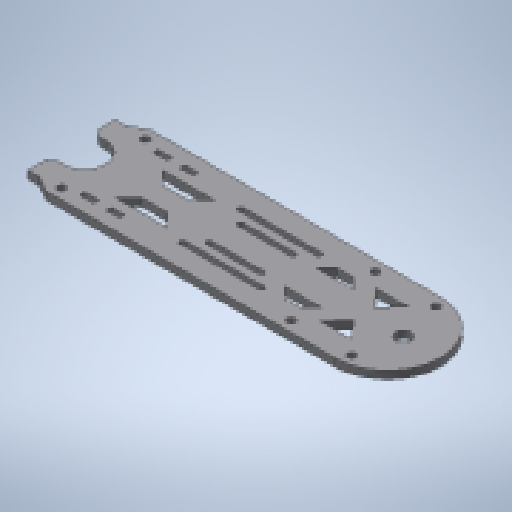
# Autodesk Inventor part: topplate.rev4
Saved by Autodesk Inventor 2025.2 (Build 292293000, 293)
## iProperties
Created: 2016-03-08
Part Number: topplate.rev4
Material: 一般
Document SubType Name: Modeling
Designer: 200288284
Density: 1 g/cm^3
Appearance: 默认值
Author: 200288284
Autodesk Inventor part; units mm, degrees
ref_plane "YZ Plane" through (0, 0, 0) normal (1, 0, 0) x (0, 1, 0)
ref_plane "XZ Plane" through (0, 0, 0) normal (0, 1, 0) x (-1, 0, 0)
ref_plane "XY Plane" through (0, 0, 0) normal (0, 0, 1) x (1, 0, 0)
sketch "Sketch1" plane through (0, 0, 0) normal (0, 1, 0) x (-1, 0, 0)
  line L0 (-71.934, -191.4381) -> (-71.9231, -191.4456)
  line L1 (19.6087, -153.4475) -> (19.6065, -153.4456)
  line L2 (-67.3897, -0.1562) -> (-37.3897, -0.1562)
  line L3 (-37.3897, 1.8438) -> (-67.3897, 1.8438)
  line L4 (-62.3897, -3.1562) -> (-42.3897, -3.1562)
  line L5 (-42.3897, -5.1562) -> (-62.3897, -5.1562)
  line L6 (-113.9275, -186.1817) -> (-113.9275, -186.2664)
  line L7 (-115.4443, -311.1974) -> (-115.4443, -311.1982)
  line L8 (-113.9275, -180.4456) -> (-113.9275, -180.5089)
  circle A0 centre (-110.3897, -10.1562) radius 3
  arc A1 (10.8743, -2.1562) -> (10.8743, -18.1562) centre (10.8743, -10.1562) ccw
  arc A2 (-42.3897, -5.1562) -> (-42.3897, -3.1562) centre (-42.3897, -4.1562) ccw
  arc A3 (-62.3897, -3.1562) -> (-62.3897, -5.1562) centre (-62.3897, -4.1562) ccw
  arc A4 (-67.3897, 1.8438) -> (-67.3897, -0.1562) centre (-67.3897, 0.8438) ccw
  arc A5 (-37.3897, -0.1562) -> (-37.3897, 1.8438) centre (-37.3897, 0.8438) ccw
  arc A6 (-104.3897, 9.8438) -> (-104.3897, -30.1562) centre (-104.3897, -10.1562) ccw
  line L9 (5.6103, 9.8438) -> (11.6725, 6.3438)
  line L10 (11.6725, 6.3438) -> (15.6725, 6.3438)
  line L11 (15.6725, 6.3438) -> (15.6725, -0.2278)
  line L12 (15.6725, -0.2278) -> (13.3743, -2.1562)
  line L13 (13.3743, -2.1562) -> (10.8743, -2.1562)
  line L14 (5.6103, 9.8438) -> (-104.3897, 9.8438)
  line L15 (-89.3897, 0.552) -> (-101.3897, 0.552)
  line L16 (-101.3897, 0.552) -> (-95.3897, -6.1562)
  line L17 (-95.3897, -6.1562) -> (-89.3897, 0.552)
  line L18 (-85.3897, -4.1562) -> (-81.3897, -0.1562)
  line L19 (-75.3897, -0.1562) -> (-71.3897, -4.1562)
  line L20 (-71.3897, -4.1562) -> (-85.3897, -4.1562)
  line L21 (-81.3897, -0.1562) -> (-75.3897, -0.1562)
  line L22 (-68.2196, -182.5089) -> (-68.232, -182.5206)
  line L23 (-104.3897, 9.8438) -> (-104.3897, -30.1562)
  line L24 (-104.3897, -10.1562) -> (10.8743, -10.1562)
  line L25 (-110.3897, -10.1562) -> (-104.3897, -10.1562)
  line L26 (10.8743, -2.1562) -> (10.8743, -18.1562)
  line L27 (5.6103, -30.1562) -> (11.6725, -26.6562)
  line L28 (11.6725, -26.6562) -> (15.6725, -26.6562)
  line L29 (15.6725, -26.6562) -> (15.6725, -20.0845)
  line L30 (15.6725, -20.0845) -> (13.3743, -18.1562)
  line L31 (13.3743, -18.1562) -> (10.8743, -18.1562)
  line L32 (5.6103, -30.1562) -> (-104.3897, -30.1562)
  line L33 (-2.3577, 2.8438) -> (-7.5577, 2.8438)
  line L34 (-7.5577, 2.8438) -> (-7.5577, 4.8438)
  line L35 (-2.3577, 4.8438) -> (-7.5577, 4.8438)
  line L36 (-2.3577, 2.8438) -> (-2.3577, 4.8438)
  line L37 (-12.3577, 2.8438) -> (-17.5577, 2.8438)
  line L38 (-17.5577, 2.8438) -> (-17.5577, 4.8438)
  line L39 (-12.3577, 4.8438) -> (-17.5577, 4.8438)
  line L40 (-12.3577, 2.8438) -> (-12.3577, 4.8438)
  line L41 (-46.7577, -10.1562) -> (-46.7577, 9.8438)
  line L42 (-2.3577, -23.1562) -> (-7.5577, -23.1562)
  line L43 (-7.5577, -23.1562) -> (-7.5577, -25.1562)
  line L44 (-2.3577, -25.1562) -> (-7.5577, -25.1562)
  line L45 (-2.3577, -23.1562) -> (-2.3577, -25.1562)
  line L46 (-12.3577, -23.1562) -> (-17.5577, -23.1562)
  line L47 (-17.5577, -23.1562) -> (-17.5577, -25.1562)
  line L48 (-12.3577, -25.1562) -> (-17.5577, -25.1562)
  line L49 (-12.3577, -23.1562) -> (-12.3577, -25.1562)
  circle A7 centre (3.6423, -25.1562) radius 1.55
  circle A8 centre (3.5423, 4.8438) radius 1.55
  circle A9 centre (-83.7577, 4.8438) radius 1.55
  circle A10 centre (-106.7577, 4.8438) radius 1.55
  circle A11 centre (-83.7577, -25.1562) radius 1.55
  circle A12 centre (-106.7577, -25.1562) radius 1.55
  line L50 (-62.3897, -17.1562) -> (-42.3897, -17.1562)
  line L51 (-42.3897, -15.1562) -> (-62.3897, -15.1562)
  line L52 (-67.3897, -20.1562) -> (-37.3897, -20.1562)
  line L53 (-37.3897, -22.1562) -> (-67.3897, -22.1562)
  arc A13 (-42.3897, -17.1562) -> (-42.3897, -15.1562) centre (-42.3897, -16.1562) ccw
  arc A14 (-62.3897, -15.1562) -> (-62.3897, -17.1562) centre (-62.3897, -16.1562) ccw
  arc A15 (-67.3897, -20.1562) -> (-67.3897, -22.1562) centre (-67.3897, -21.1562) ccw
  arc A16 (-37.3897, -22.1562) -> (-37.3897, -20.1562) centre (-37.3897, -21.1562) ccw
  line L54 (-89.3897, -20.8644) -> (-101.3897, -20.8644)
  line L55 (-101.3897, -20.8644) -> (-95.3897, -14.1562)
  line L56 (-95.3897, -14.1562) -> (-89.3897, -20.8644)
  line L57 (-85.3897, -16.1562) -> (-81.3897, -20.1562)
  line L58 (-75.3897, -20.1562) -> (-71.3897, -16.1562)
  line L59 (-71.3897, -16.1562) -> (-85.3897, -16.1562)
  line L60 (-81.3897, -20.1562) -> (-75.3897, -20.1562)
  line L61 (-29.7577, -1.1562) -> (-9.7577, -1.1562)
  line L62 (-9.7577, -1.1562) -> (-14.7577, -6.1562)
  line L63 (-14.7577, -6.1562) -> (-24.7577, -6.1562)
  line L64 (-24.7577, -6.1562) -> (-29.7577, -1.1562)
  line L65 (-29.7577, -19.1562) -> (-9.7577, -19.1562)
  line L66 (-9.7577, -19.1562) -> (-14.7577, -14.1562)
  line L67 (-14.7577, -14.1562) -> (-24.7577, -14.1562)
  line L68 (-24.7577, -14.1562) -> (-29.7577, -19.1562)
  dimension "d39" = 6
  dimension "d54" = 40
  dimension "d55" = 6
  dimension "d56" = 20
  dimension "d58" = 110
  dimension "d60" = 150
  dimension "d61" = 130
  dimension "d62" = 4
  dimension "d63" = 2.5
  dimension "d64" = 7
  dimension "d65" = 3
  dimension "d70" = 8
  dimension "d74" = 2
  dimension "d75" = 5.2
  dimension "d76" = 2
  dimension "d77" = 5.2
  dimension "d78" = 4.8
  dimension "d79" = 13
  dimension "d80" = 13
  dimension "d81" = 29.2
  dimension "d82" = 3.1
  dimension "d83" = 3.1
  dimension "d84" = 5.9
  dimension "d85" = 6
  dimension "d86" = 15
  dimension "d87" = 15
  dimension "d88" = 3.1
  dimension "d89" = 3.1
  dimension "d90" = 15
  dimension "d91" = 15
  dimension "d92" = 37
  dimension "d93" = 23
  dimension "d94" = 12
  dimension "d95" = 9
  dimension "d96" = 14
  dimension "d97" = 6
  dimension "d99" = 4
  dimension "d100" = 9
  dimension "d101" = 6
  dimension "d102" = 10
  dimension "d103" = 2
  dimension "d104" = 20
  dimension "d105" = 2
  dimension "d106" = 5
  dimension "d108" = 30
  dimension "d109" = 10
  dimension "d110" = 42
  dimension "d111" = 5
  dimension "d112" = 20
  dimension "d113" = 10
  dimension "d114" = 45
  dimension "d115" = 4
  dimension "d116" = 22
  constraints: 138 end point, 38 symmetric about line, 20 point on circle, 17 centre point, 8 horizontal, 8 tangent, 6 perpendicular, 4 parallel, 3 midpoint, 2 equal length, 2 vertical, 1 point on line, 7 other
  measures "d39" diameter of A0
  measures "d54" distance of L14.end L23.end
  measures "d55" distance of L25.start L24.start
  measures "d56" radius of A6
  measures "d58" distance of L9.start L14.end
  measures "d60" angle of L9 L14
  measures "d61" angle of L11 L12
  measures "d62" distance of L9.end L10.end
  measures "d63" distance of L12.end L13.end
  measures "d64" distance of L9.start L9.end
  measures "d65" distance of L11.end L12.end
  measures "d70" radius of A1
  measures "d74" distance between parallel lines of L37 L39
  measures "d75" distance between parallel lines of L40 L38
  measures "d76" distance between parallel lines of L35 L33
  measures "d77" distance between parallel lines of L36 L34
  measures "d78" distance between parallel lines of L40 L34
  measures "d79" distance between parallel lines of L24 L33
  measures "d80" distance between parallel lines of L24 L37
  measures "d81" distance between parallel lines of L38 L41
  measures "d82" diameter of A7
  measures "d83" diameter of A8
  measures "d84" distance from line of L36 A8.centre
  measures "d85" distance from line of L45 A7.centre
  measures "d86" distance from line of L24 A7.centre
  measures "d87" distance from line of L24 A8.centre
  measures "d88" diameter of A10
  measures "d89" diameter of A9
  measures "d90" distance from line of L24 A10.centre
  measures "d91" distance from line of A9.centre L24
  measures "d92" distance from line of L41 A9.centre
  measures "d93" distance of A10.centre A9.centre
  measures "d94" distance of L15.start L15.end
  measures "d95" distance of L15.end L16.end
  measures "d96" distance of L19.end L18.start
  measures "d97" distance of L18.end L19.start
  measures "d99" distance from line of L24 L16.end
  measures "d100" distance from line of L23 L16.end
  measures "d101" distance between parallel lines of L24 L20
  measures "d102" horizontal distance of L16.end L18.start
  measures "d103" distance between parallel lines of L4 L5
  measures "d104" distance of L5.start L5.end
  measures "d105" distance between parallel lines of L3 L2
  measures "d106" distance between parallel lines of L5 L24
  measures "d108" distance of L2.start L2.end
  measures "d109" distance between parallel lines of L24 L2
  measures "d110" distance from line of L23 A3.centre
  measures "d111" horizontal distance of A3.centre A4.centre
  measures "d112" distance of L61.start L61.end
  measures "d113" distance of L62.end L63.end
  measures "d114" angle of L61 L64
  measures "d115" distance between parallel lines of L63 L24
  measures "d116" distance from line of L41 L63.end
extrude "Extrusion1" add sketch "Sketch1" along normal blind 3 contours L2 L41 L4 A3 L5 L24 L23 L14 L3 A4 | L2 A5 L3 L41 L14 L9 L10 L11 L12 L13 A1 L24 L5 A2 L4 | L24 A1 L31 L30 L29 L28 L27 L32 L23 | L23 A6
body "Solid1"
